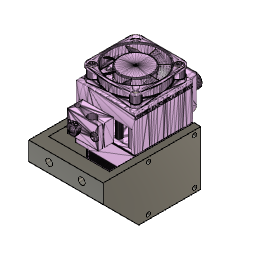
Hemera bowden mount v1 (Autodesk Fusion 360 design; units mm, degrees)
Autodesk Fusion 360 part; units mm, degrees
mesh "Mesh1" [no effect]
ref_plane "WorkPlane1" through (2.38, 0, 0) normal (1, 0, 0) x (0, 1, 0)
ref_plane "WorkPlane2" through (46.385, 0, 0) normal (1, 0, 0) x (0, 1, 0)
sketch "Sketch2" plane through (46.385, 0, 0) normal (1, 0, 0) x (0, 1, 0)
  line L0 (63.2389, 40.7601) -> (-3.7611, 40.7601)
  line L1 (-3.7611, 40.7601) -> (-3.7611, 27.7601)
  line L2 (-3.7611, 27.7601) -> (63.2389, 27.7601)
  line L3 (63.2389, 27.7601) -> (63.2389, 40.7601)
  circle A0 centre (24.6228, 37.4955) radius 1.52
  circle A1 centre (58.6228, 37.4955) radius 1.52
  line L4 (63.2389, 27.7601) -> (20, 27.7601)
  line L5 (20, 27.7601) -> (20, -1)
  line L6 (20, -1) -> (63.2389, -1)
  line L7 (63.2389, -1) -> (63.2389, 27.7601)
  circle A2 centre (58.6228, 3.9955) radius 1.52
  circle A3 centre (24.6228, 3.9955) radius 1.52
  dimension "d6" = 67
  dimension "d7" = 13
  dimension "d8" = 3.04
  dimension "d9" = 3.04
  dimension "d14" = 3.04
  dimension "d15" = 3.04
  constraint horizontal L0
  constraint vertical L1
  constraint horizontal L2
  constraint vertical L3
  constraint horizontal L4
  constraint vertical L5
  constraint horizontal L6
  constraint vertical L7
  measures "d6" distance of L1.end L2.end
  measures "d7" distance of L0.end L1.end
  measures "d8" diameter of A0
  measures "d9" diameter of A1
  measures "d14" diameter of A3
  measures "d15" diameter of A2
sketch "Sketch3" plane through (2.38, 0, 0) normal (1, 0, 0) x (0, 1, 0)
  line L0 (-3.7611, 40.7601) -> (-3.7611, 27.7601)
  line L1 (63.2389, 27.7601) -> (63.2389, 40.7601)
  line L2 (63.2389, -1) -> (63.2389, 27.7601)
  line L3 (20, 27.7601) -> (20, -1)
  line L4 (20, -1) -> (63.2389, -1)
  line L5 (-3.7611, 27.7601) -> (63.2389, 27.7601)
  line L6 (63.2389, 40.7601) -> (-3.7611, 40.7601)
  line L7 (63.2389, 27.7601) -> (20, 27.7601)
  circle A0 centre (58.6228, 37.4955) radius 1.52
  circle A1 centre (24.6228, 37.4955) radius 1.52
  circle A2 centre (58.6228, 3.9955) radius 1.52
  circle A3 centre (24.6228, 3.9955) radius 1.52
  dimension "d10" = 67
  dimension "d11" = 13
  dimension "d12" = 3.04
  dimension "d13" = 3.04
  dimension "d16" = 3.04
  dimension "d17" = 3.04
  constraint horizontal L6
  constraint vertical L0
  constraint horizontal L5
  constraint vertical L1
  constraint horizontal L7
  constraint vertical L3
  constraint horizontal L4
  constraint vertical L2
  measures "d10" distance of L0.end L1.start
  measures "d11" distance of L0.start L0.end
  measures "d12" diameter of A1
  measures "d13" diameter of A0
  measures "d16" diameter of A3
  measures "d17" diameter of A2
extrude "Extrude1" add sketch "Sketch3" against normal blind 5 makes body 1
extrude "Extrude2" add sketch "Sketch2" along normal blind 5 separate body makes body 2
sketch "Sketch4" plane through (0, -3.7611, 0) normal (0, -1, 0) x (1, 0, 0)
  line L0 (2.38, 27.7601) -> (2.38, 40.7601)
  line L1 (2.38, 40.7601) -> (-2.62, 40.7601)
  line L2 (-2.62, 40.7601) -> (-2.62, 27.7601)
  line L3 (-2.62, 27.7601) -> (2.38, 27.7601)
  line L4 (-2.62, 40.7601) -> (51.385, 40.7601)
  line L5 (51.385, 40.7601) -> (51.385, 27.76)
  line L6 (51.385, 27.76) -> (-2.62, 27.76)
  line L7 (-2.62, 27.76) -> (-2.62, 40.7601)
  constraint horizontal L4
  constraint vertical L5
  constraint horizontal L6
  constraint vertical L7
  constraint coincident L1.end L2.start
extrude "Extrude3" add sketch "Sketch4" along normal blind 5 bodies 1 2
extrude "Extrude4" cut 2 faces at (48.0517, 20, 18.1734) (0.7133, 20, 18.1734) along direction (0, -1, 0) blind 28.75 on bodies 1 bodies 1
extrude "Extrude5" add 2 faces at (48.0517, 20, 18.1734) (0.7133, 20, 18.1734) along direction (0, -1, 0) blind 28.75 on bodies 1 bodies 1
chamfer "Chamfer1" distance 28 angle 45 2 edges at (48.885, -8.75, -1) (-0.12, -8.75, -1) on bodies 1
sketch "Sketch5" plane through (0, -8.7611, 0) normal (0, -1, 0) x (1, 0, 0)
  line L0 (-2.62, 27.76) -> (51.385, 27.76)
  line L1 (51.385, 27.76) -> (51.385, 40.7601)
  line L2 (51.385, 40.7601) -> (-2.62, 40.7601)
  line L3 (-2.62, 40.7601) -> (-2.62, 27.76)
  circle A0 centre (12, 34) radius 2.5
  circle A1 centre (36, 34) radius 2.5
  dimension "d29" = 5
  dimension "d30" = 5
  measures "d29" diameter of A0
  measures "d30" diameter of A1
extrude "Extrude6" add 1 faces at (31.7167, -3.7611, 32.0934) along direction (0, 1, 0) blind 4.6 on bodies 1 bodies 1
sketch "Sketch6" plane through (0, 0.8389, 0) normal (0, 1, 0) x (-1, 0, 0)
  line L0 (-46.385, 40.7601) -> (-46.385, 27.76)
  line L1 (-46.385, 27.76) -> (-2.38, 27.76)
  line L2 (-2.38, 27.76) -> (-2.38, 40.7601)
  line L3 (-2.38, 40.7601) -> (-46.385, 40.7601)
  circle A0 centre (-36, 34) radius 3.75
  circle A1 centre (-12, 34) radius 3.75
  dimension "d33" = 7.5
  dimension "d34" = 7.5
  measures "d33" diameter of A0
  measures "d34" diameter of A1
extrude "Extrude7" cut sketch "Sketch6" against normal blind 4.5 contours A0 | A1 bodies 1
extrude "Extrude8" cut sketch "Sketch5" against normal blind 16 contours A0 | A1 bodies 1
sketch "Sketch7" plane through (0, 0, -1) normal (0, 0, -1) x (1, 0, 0)
  line L0 (51.385, -19.25) -> (46.385, -19.25)
  line L1 (46.385, -19.25) -> (46.385, -63.2389)
  line L2 (46.385, -63.2389) -> (51.385, -63.2389)
  line L3 (51.385, -63.2389) -> (51.385, -19.25)
  line L4 (51.385, -63.2389) -> (-2.6185, -63.2389)
  line L5 (-2.6185, -63.2389) -> (-2.6185, -19.2527)
  line L6 (-2.6185, -19.2527) -> (51.385, -19.2527)
  line L7 (51.385, -19.2527) -> (51.385, -63.2389)
  constraint horizontal L4
  constraint vertical L5
  constraint horizontal L6
  constraint vertical L7
  constraint coincident L2.end L3.start
extrude "Extrude9" [suppressed]
extrude "Extrude10" add 2 faces at (31.7167, -5.5537, 27.7601) (-0.9533, -8.7537, 27.7601) along direction (0, 0, -1) blind 1 on bodies 1 bodies 1
chamfer "Chamfer2" distance 0.2 angle 45 1 edges at (24.3825, -8.7611, 26.76) on bodies 1
extrude "Extrude11" cut 1 faces at (47.09, -8.7611, 33.9067) along direction (0, 1, 0) blind 0.01 on bodies 1 bodies 1
extrude "Extrude12" add 1 faces at (17.0483, -5.3937, 26.7601) along direction (0, 0, -1) blind 5 on bodies 1 bodies 1
chamfer "Chamfer3" distance 5 angle 45 1 edges at (24.3825, -8.5611, 21.76) on bodies 1
extrude "Extrude13" cut 2 faces at (49.7183, 2.33, 15.92) (-0.9533, 2.33, 15.92) along direction (0, -0.707107, -0.707107) blind 0.01 on bodies 1 bodies 1
extrude "Extrude14" cut 1 faces at (2.38, 46.9102, 15.4982) along direction (-1, 0, 0) blind 0.4 on bodies 1 bodies 1
extrude "Extrude15" cut 1 faces at (46.385, 46.9102, 15.4982) along direction (1, 0, 0) blind 0.4 on bodies 1 bodies 1
extrude "Extrude16" add 1 faces at (-2.62, 12.9229, 22.8304) along direction (-1, 0, 0) blind 0.4 on bodies 1 bodies 1
extrude "Extrude17" add 1 faces at (51.385, 12.9229, 22.8304) along direction (1, 0, 0) blind 0.4 on bodies 1 bodies 1
extrude "Extrude18" cut 2 faces at (50.1183, 48.5759, -1) (-1.3533, 33.913, -1) along direction (0, 0, 1) blind 1.75 on bodies 1 bodies 1
sketch "Sketch8" plane through (-3.02, 0, 0) normal (-1, 0, 0) x (0, -1, 0)
  line L0 (-19.25, 0.75) -> (-19.25, -1)
  line L1 (-19.25, -1) -> (8.75, 27)
  line L2 (8.75, 27) -> (8.7511, 26.9989)
  line L3 (8.7511, 26.9989) -> (8.7511, 40.7601)
  line L4 (8.7511, 40.7601) -> (-63.2389, 40.7601)
  line L5 (-63.2389, 40.7601) -> (-63.2389, 0.75)
  line L6 (-63.2389, 0.75) -> (-19.25, 0.75)
  circle A0 centre (-24.6228, 3.9955) radius 1.52
  circle A1 centre (-58.6228, 37.4955) radius 1.52
  circle A2 centre (-24.6228, 37.4955) radius 1.52
  circle A3 centre (-58.6228, 3.9955) radius 1.52
  line L7 (-19.25, 0.75) -> (-16.6, 0.75)
  line L8 (-16.6, 0.75) -> (-16.6, -1.1)
  line L9 (-16.6, -1.1) -> (-19.25, -1.1)
  line L10 (-19.25, -1.1) -> (-19.25, 0.75)
  constraint horizontal L7
  constraint vertical L8
  constraint horizontal L9
  constraint vertical L10
  constraint coincident L0.start L6.end
extrude "Extrude19" cut sketch "Sketch8" against normal blind 114 contours L0 L1 L7 L10 | L1 L7 L8 L9 L10 bodies 1
named bodies: "EXTRUDER MOUNT"
